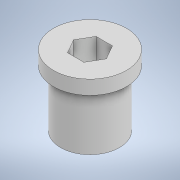
# Autodesk Inventor part: Climber Axel End Cap
Saved by Autodesk Inventor 2020 (Build 240168000, 168)
## iProperties
Created: 2020-02-03
Part Number: Climber Axel End Cap
Material: Generic
Document SubType Name: Modeling
Designer: JimAndVal
Density: 1 g/cm^3
Appearance: Default
Author: JimAndVal
Autodesk Inventor part; units mm, degrees
ref_plane "YZ Plane" through (0, 0, 0) normal (1, 0, 0) x (0, 1, 0)
ref_plane "XZ Plane" through (0, 0, 0) normal (0, 1, 0) x (-1, 0, 0)
ref_plane "XY Plane" through (0, 0, 0) normal (0, 0, 1) x (1, 0, 0)
sketch "Sketch1" plane through (0, 0, 0) normal (0, 0, 1) x (1, 0, 0)
  line L0 (0, 0) -> (0, 31.75)
  line L1 (0, 31.75) -> (0.7288, 31.75)
  line L2 (16.4465, 31.75) -> (16.4465, 25.4)
  line L3 (16.4465, 25.4) -> (13.2715, 25.4)
  line L4 (13.2715, 25.4) -> (13.2715, 0)
  line L5 (13.2715, 0) -> (0, 0)
  line L6 (16.4465, 31.75) -> (0.7288, 31.75)
  dimension "d0" = 13.2715
  dimension "d1" = 31.75
  dimension "d2" = 25.4
  dimension "d4" = 3.175
  constraints: 14 end point, 4 perpendicular, 2 vertical, 1 horizontal, 1 point on line
  measures "d0" distance of L4.end L0.start
  measures "d1" distance of L0.start L0.end
  measures "d2" vertical distance of L4.end L2.end
  measures "d4" distance of L2.end L3.end
revolve "Revolution1" add sketch "Sketch1" angle 360 about axis through (0, 0, 0) along (0, 1, 0)
sketch "Sketch2" plane through (0, 31.75, 0) normal (0, 1, 0) x (1, 0, 0)
  circle A0 centre (0, 0) radius 6.4135 construction
  line L0 (7.4056, -0.019) -> (3.6864, -6.423)
  line L1 (3.6864, -6.423) -> (-3.7193, -6.404)
  line L2 (-3.7193, -6.404) -> (-7.4056, 0.019)
  line L3 (-7.4056, 0.019) -> (-3.6864, 6.423)
  line L4 (-3.6864, 6.423) -> (3.7193, 6.404)
  line L5 (3.7193, 6.404) -> (7.4056, -0.019)
  point P0 (5.5625, 3.1925)
  dimension "d5" = 12.827
  constraints: 12 end point, 2 coincident, 1 midpoint, 16 other
extrude "Extrusion1" cut sketch "Sketch2" against normal through all
body "Solid1"
